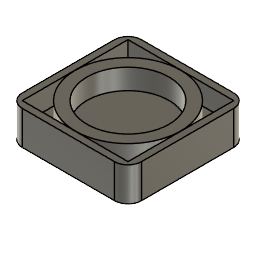
에어스프링_어댑터2 (Autodesk Fusion 360 design; units mm, degrees)
Autodesk Fusion 360 part; units mm, degrees
sketch "스케치1" plane through (0, 0, 0) normal (0, 0, 1) x (1, 0, 0)
  line L0 (0, 0) -> (78, 0)
  line L1 (78, 0) -> (78, -78)
  line L2 (78, -78) -> (0, -78)
  line L3 (0, -78) -> (0, 0)
  line L4 (83, -83) -> (-5, -83)
  line L5 (-5, -83) -> (-5, 5)
  line L6 (-5, 5) -> (83, 5)
  line L7 (83, 5) -> (83, -83)
  dimension "d1" = 78
  dimension "d2" = 78
  dimension "d3" = -5
  constraint horizontal L0
  constraint vertical L1
  constraint horizontal L2
  constraint vertical L3
  constraint coincident L0.start L3.end
  measures "d1" distance of L0.start L0.end
  measures "d2" distance of L0.end L1.end
extrude "돌출1" add sketch "스케치1" along normal blind 15 makes body 1
extrude "돌출2" add sketch "스케치1" against normal blind 10 contours L0 L1 L2 L3 | L4 L5 L6 L7 bodies 1
sketch "스케치2" plane through (0, 0, -10) normal (0, 0, -1) x (1, 0, 0)
  line L0 (-5, -5) -> (83, -5)
  line L1 (83, -5) -> (83, 83)
  line L2 (83, 83) -> (-5, 83)
  line L3 (-5, 83) -> (-5, -5)
  circle A0 centre (39, 39) radius 15.05
  circle A1 centre (39, 39) radius 25.05
  dimension "d8" = 30.1
  dimension "d9" = 10
  measures "d8" diameter of A0
extrude "돌출3" add sketch "스케치2" along normal blind 10 contours A1 bodies 1
fillet "필렛1" radius 10 4 edges at (-5, 5, 2.5) (83, 5, 2.5) (83, -83, 2.5) (-5, -83, 2.5) on bodies 1
fillet "필렛2" radius 10 1 edges at (15.6452, -48.0585, -10) on bodies 1
sketch "스케치3" plane through (0, 0, 0) normal (0, 0, 1) x (-1, 0, 0)
  line L0 (-78, 78) -> (-78, 0)
  line L1 (-78, 0) -> (0, 0)
  line L2 (0, 0) -> (0, 78)
  line L3 (0, 78) -> (-78, 78)
  circle A0 centre (-39, 39) radius 30.25
  line L4 (-0.12, 77.88) -> (-77.88, 77.88)
  line L5 (-77.88, 77.88) -> (-77.88, 0.12)
  line L6 (-77.88, 0.12) -> (-0.12, 0.12)
  line L7 (-0.12, 0.12) -> (-0.12, 77.88)
  dimension "d16" = 60.5
  dimension "d17" = -0.12
  measures "d16" diameter of A0
extrude "돌출4" add sketch "스케치3" along normal blind 15 separate body contours L4 L5 L6 L7 makes body 2
sketch "스케치4" plane through (0, 0, 15) normal (0, 0, 1) x (-1, 0, 0)
  circle A0 centre (-39, 39) radius 30.25
  line L0 (-0.12, 0.12) -> (-0.12, 77.88)
  line L1 (-0.12, 77.88) -> (-77.88, 77.88)
  line L2 (-77.88, 77.88) -> (-77.88, 0.12)
  line L3 (-77.88, 0.12) -> (-0.12, 0.12)
  circle A1 centre (-39, 39) radius 30
  dimension "d20" = 60
  constraint concentric A0 A1
  measures "d20" diameter of A1
extrude "돌출6" add sketch "스케치4" along normal blind 20 from surface at -15 separate body contours A1 makes body 3
fillet "필렛3" radius 10 4 edges at (0.12, -0.12, 7.5) (0.12, -77.88, 7.5) (77.88, -0.12, 7.5) (77.88, -77.88, 7.5) on bodies 2
sketch "스케치5" plane through (0, 0, 15) normal (0, 0, 1) x (-1, 0, 0)
  circle A0 centre (-39, 39) radius 30.25
  arc A1 (-67.88, 77.88) -> (-77.88, 67.88) centre (-67.88, 67.88) ccw
  line L0 (-77.88, 67.88) -> (-77.88, 10.12)
  arc A2 (-77.88, 10.12) -> (-67.88, 0.12) centre (-67.88, 10.12) ccw
  line L1 (-67.88, 0.12) -> (-10.12, 0.12)
  arc A3 (-10.12, 0.12) -> (-0.12, 10.12) centre (-10.12, 10.12) ccw
  line L2 (-0.12, 10.12) -> (-0.12, 67.88)
  arc A4 (-0.12, 67.88) -> (-10.12, 77.88) centre (-10.12, 67.88) ccw
  line L3 (-10.12, 77.88) -> (-67.88, 77.88)
  line L4 (-39, 77.88) -> (-39, -15)
  line L5 (-39, 39) -> (-115, 39)
  line L6 (-115, 39) -> (21.9239, 39)
  line L7 (-8.5, 89) -> (-69.5, 89)
  line L8 (-69.5, 89) -> (-69.5, -11)
  line L9 (-69.5, -11) -> (-8.5, -11)
  line L10 (-8.5, -11) -> (-8.5, 89)
  line L11 (-8.5, 89) -> (-69.5, -11) construction
  line L12 (-69.5, 89) -> (-8.5, -11) construction
  line L13 (-103.3852, 8.5) -> (25.3852, 8.5)
  line L14 (25.3852, 8.5) -> (25.3852, 69.5)
  line L15 (25.3852, 69.5) -> (-103.3852, 69.5)
  line L16 (-103.3852, 69.5) -> (-103.3852, 8.5)
  line L17 (-103.3852, 8.5) -> (25.3852, 69.5) construction
  line L18 (25.3852, 8.5) -> (-103.3852, 69.5) construction
  circle A5 centre (-39, 39) radius 38.88
  point P0 (-39, 39)
  point P1 (-39, 39)
  dimension "d28" = 100
  dimension "d29" = 61
  dimension "d30" = 61
  constraint midpoint L3 L4.start
  constraint perpendicular L1 L4
  constraint coincident P0 A0.centre
  constraint perpendicular L4 L5
  constraint perpendicular L2 L6
  constraint horizontal L7
  constraint perpendicular L7 L8
  constraint parallel L7 L9
  constraint parallel L8 L10
  constraint coincident L11 P1
  constraint coincident L12 P1
  constraint horizontal L13
  constraint perpendicular L13 L14
  constraint parallel L13 L15
  constraint parallel L14 L16
  constraint coincident L17 P1
  constraint coincident L18 P1
  constraint coincident P1 P0
  constraint coincident L4.start A5
  measures "d28" distance of L7.end L8.end
  measures "d29" distance of L7.start L7.end
  measures "d30" distance of L13.end L14.end
extrude "돌출7" cut sketch "스케치5" against normal blind 35 contours L2 A4 L10 L15 A5 | A3 L2 L10 L13 A5 | L10 L13 A5 | L10 L15 A5 | A1 L3 L8 L15 A5 | A4 L3 L10 L15 A5 | L8 L15 A5 | L1 A3 L10 L13 A5 | A2 L1 L8 L13 A5 | L8 L13 A5 | A3 L10 L13 | A4 L10 L15 | L0 A2 L8 L13 A5 | A1 L0 L8 L15 A5 | A1 L8 L15 | A2 L8 L13 bodies 2
extrude "돌출5" [rolled back] along distance 20 taper angle 0
hidden bodies 3
named bodies: "에어스프링 어댑터", "에어스프링 모델"
